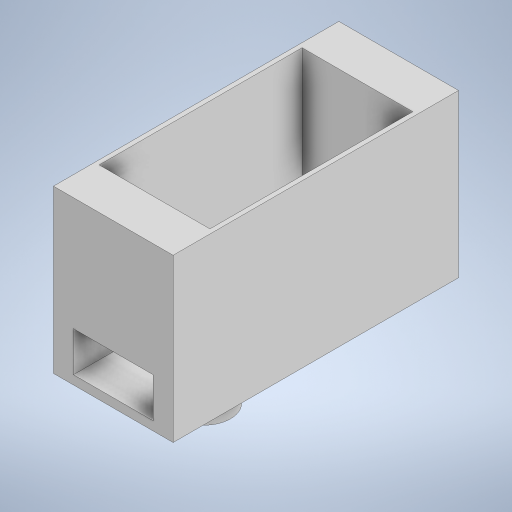
# Autodesk Inventor part: Servo Top Mount
Saved by Autodesk Inventor 2023 (Build 270158000, 158)
## iProperties
Created: 2022-10-13
Part Number: Servo Top Mount
Material: Generic
Document SubType Name: Modeling
Designer: GROS
Density: 1 g/cm^3
Appearance: Default
Author: GROS
Autodesk Inventor part; units mm, degrees
ref_plane "YZ Plane" through (0, 0, 0) normal (1, 0, 0) x (0, 1, 0)
ref_plane "XZ Plane" through (0, 0, 0) normal (0, 1, 0) x (-1, 0, 0)
ref_plane "XY Plane" through (0, 0, 0) normal (0, 0, 1) x (1, 0, 0)
sketch "Sketch1" plane through (0, 0, 0) normal (0, 1, 0) x (-1, 0, 0)
  line L0 (0, 0) -> (12.5, 0)
  line L1 (12.5, 0) -> (12.5, -22.9)
  line L2 (12.5, -22.9) -> (0, -22.9)
  line L3 (0, -22.9) -> (0, 0)
  line L4 (12.5, 0) -> (13, 0)
  line L5 (0, -22.9) -> (-0.5, -22.9)
  line L6 (13, 0) -> (13, 4.65)
  line L7 (-0.5, -22.9) -> (-0.5, -27.55)
  line L8 (13, 4.65) -> (-0.5, 4.65)
  line L9 (-0.5, 4.65) -> (-0.5, -27.55)
  line L10 (-0.5, -27.55) -> (13, -27.55)
  line L11 (13, -27.55) -> (13, 4.65)
  line L12 (6.25, 0) -> (6.25, 2.45)
  line L13 (6.25, -22.9) -> (6.25, -25.35)
  circle A0 centre (6.25, 2.45) radius 0.75
  circle A1 centre (6.25, -25.35) radius 0.75
  dimension "d0" = 12.5
  dimension "d1" = 22.9
  dimension "d2" = 0.5
  dimension "d3" = 0.5
  dimension "d4" = 4.65
  dimension "d5" = 4.65
  dimension "d6" = 2.45
  dimension "d7" = 2.45
  dimension "d8" = 1.5
  dimension "d9" = 1.5
  constraints: 28 end point, 4 horizontal, 4 parallel, 4 vertical, 2 centre point, 2 coincident, 2 midpoint, 2 perpendicular
  measures "d0" distance of L1.end L2.end
  measures "d1" distance of L0.end L1.end
  measures "d2" distance of L2.end L5.end
  measures "d3" distance of L0.end L4.end
  measures "d4" distance of L4.end L6.end
  measures "d5" distance of L5.end L7.end
  measures "d6" distance of L13.start L13.end
  measures "d7" distance of L12.start L12.end
  measures "d8" diameter of A1
  measures "d9" diameter of A0
extrude "Extrusion1" add sketch "Sketch1" along normal blind 17.3 contours A0 | L3 L5 L9 L8 L6 L4 L0 | A1 | L2 L1 L4 L11 L10 L7 L5
extrude "Extrusion2" add sketch "Sketch1" against normal blind 1 contours A0 | L3 L5 L9 L8 L6 L4 L0 | L0 L1 L2 L3 | A1 | L2 L1 L4 L11 L10 L7 L5
sketch "Sketch2" plane through (0, -1, 0) normal (0, -1, 0) x (1, 0, 0)
  line L0 (0.5, 4.65) -> (0.5, -27.55) projected
  line L1 (-12.5, -22.9) -> (0, -22.9) projected
  line L2 (-13, -27.55) -> (-13, 4.65) projected
  line L3 (-13, 4.65) -> (-13, 0)
  line L4 (-13, 0) -> (-6.3, 0)
  line L5 (0, 0) -> (-12.5, 0) projected
  line L6 (-6.3, 0) -> (-6.3, -5.6)
  circle A0 centre (-6.3, -5.6) radius 3.025
  dimension "d20" = 4.65
  dimension "d21" = 6.7
  dimension "d22" = 5.6
  dimension "d23" = 6.05
  constraints: 6 end point, 2 point on line, 1 centre point, 1 coincident, 1 vertical
  measures "d20" distance of L2.end L3.end
  measures "d21" distance of L3.end L4.end
  measures "d22" distance of L4.end L6.end
  measures "d23" diameter of A0
extrude "Extrusion3" add sketch "Sketch2" along normal blind 4.7
sketch "Sketch3" plane through (-6.3, -5.7, -5.6) normal (0, -1, 0) x (1, 0, 0)
  line L0 (0, 0) -> (1.385, 0)
  line L1 (0, 0) -> (0, 1.385)
  line L2 (1.385, 0) -> (1.385, 0.32)
  line L3 (0, 1.385) -> (-0.32, 1.385)
  line L4 (-0.32, 1.385) -> (0.32, 1.385)
  line L5 (0.32, 1.385) -> (0.32, -1.385)
  line L6 (0.32, -1.385) -> (-0.32, -1.385)
  line L7 (-0.32, -1.385) -> (-0.32, 1.385)
  line L8 (1.385, 0.32) -> (-1.385, 0.32)
  line L9 (-1.385, 0.32) -> (-1.385, -0.32)
  line L10 (-1.385, -0.32) -> (1.385, -0.32)
  line L11 (1.385, -0.32) -> (1.385, 0.32)
  point P0 (6.3, 5.6)
  point P1 (-0.32, 0.32)
  point P2 (-0.32, -0.32)
  point P3 (0.32, -0.32)
  point P4 (0.32, 0.32)
  dimension "d24" = 1.385
  dimension "d25" = 1.385
  dimension "d26" = 0.32
  dimension "d27" = 0.32
  dimension "d28" = 0.64
  dimension "d30" = 2.77
  dimension "d31" = 0.64
  dimension "d32" = 2.77
  constraints: 24 end point, 4 horizontal, 4 parallel, 2 perpendicular, 2 vertical
  measures "d24" distance of L0.start L1.end
  measures "d25" distance of L0.start L0.end
  measures "d26" distance of L1.end L3.end
  measures "d27" distance of L0.end L2.end
  measures "d28" distance of L3.end L4.end
  measures "d30" distance of L4.end L5.end
  measures "d31" distance of L10.end L2.end
  measures "d32" distance of L9.end L10.end
extrude "Extrusion4" [suppressed]
sketch "Sketch7" plane through (-13, 17.3, 4.65) normal (0, 0, 1) x (1, 0, 0)
  line L0 (0, -18.3) -> (13.5, -18.3) projected
  line L1 (6.75, -18.3) -> (6.75, -17.3)
  line L2 (6.75, -17.3) -> (2.25, -17.3)
  line L3 (0.5, -17.3) -> (13, -17.3) projected
  line L4 (2.25, -17.3) -> (11.25, -17.3)
  line L5 (11.25, -17.3) -> (11.25, -12.8)
  line L6 (11.25, -12.8) -> (2.25, -12.8)
  line L7 (2.25, -12.8) -> (2.25, -17.3)
  dimension "d47" = 1
  dimension "d48" = 4.5
  dimension "d49" = 4.5
  dimension "d50" = 9
  constraints: 12 end point, 2 parallel, 1 horizontal, 1 midpoint, 1 perpendicular, 1 point on line, 1 vertical
  measures "d47" distance of L1.start L1.end
  measures "d48" distance of L1.end L2.end
  measures "d49" distance of L6.end L2.end
  measures "d50" distance of L5.end L6.end
extrude "Extrusion7" cut sketch "Sketch7" against normal up to next
sketch "Sketch8" plane through (-6.3, -5.7, -5.6) normal (0, -1, 0) x (1, 0, 0)
  line L0 (0, 0) -> (0, 1.7)
  line L1 (0, 1.7) -> (0.37, 1.7)
  line L2 (0.37, 1.7) -> (0.37, -1.7)
  line L3 (0.37, -1.7) -> (-0.37, -1.7)
  line L4 (-0.37, -1.7) -> (-0.37, 1.7)
  line L5 (-0.37, 1.7) -> (0, 1.7)
  line L6 (0, 0) -> (1.2021, -1.2021)
  line L7 (1.2021, -1.2021) -> (0.9405, -1.4637)
  line L8 (0.9405, -1.4637) -> (-1.4637, 0.9405)
  line L9 (-1.4637, 0.9405) -> (-0.9405, 1.4637)
  line L10 (-0.9405, 1.4637) -> (1.4637, -0.9405)
  line L11 (1.4637, -0.9405) -> (1.2021, -1.2021)
  point P0 (6.3, 5.6)
  dimension "d53" = 1.7
  dimension "d54" = 0.37
  dimension "d55" = 3.4
  dimension "d56" = 0.74
  dimension "d57" = 3.4
  dimension "d60" = 1.7
  dimension "d61" = 0.37
  dimension "d62" = 3.4
  dimension "d63" = 0.74
  dimension "d64" = 3.4
  constraints: 24 end point, 3 vertical, 2 horizontal
  measures "d53" distance of L0.start L0.end
  measures "d54" distance of L0.end L1.end
  measures "d55" distance of L1.end L2.end
  measures "d56" distance of L2.end L3.end
  measures "d57" distance of L3.end L4.end
  measures "d60" distance of L6.start L6.end
  measures "d61" distance of L6.end L7.end
  measures "d62" distance of L7.end L8.end
  measures "d63" distance of L8.end L9.end
  measures "d64" distance of L9.end L10.end
extrude "Extrusion8" cut sketch "Sketch8" against normal blind 3 contours L6 L2 L8 L4 L10 L0 | L0 L10 L2 L6 | L6 L7 L8 L2 | L2 L10 L11 L6 | L4 L8 L9 L10
body "Solid1"
